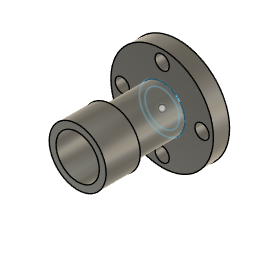
3D Plancha 1 (Autodesk Fusion 360 design; units mm, degrees)
Autodesk Fusion 360 part; units mm, degrees
sketch "Boceto1" plane through (0, 0, 0) normal (0, 1, 0) x (1, 0, 0)
  circle A0 centre (70, 0) radius 45
extrude "Extruir2" add sketch "Boceto1" along normal blind 14.2 makes body 1
sketch "Boceto2" plane through (0, 0, 0) normal (0, 1, 0) x (1, 0, 0)
  circle A0 centre (70, -35) radius 6.25
  circle A1 centre (35, 0) radius 6.25
  circle A2 centre (70, 35) radius 6.25
  circle A3 centre (105, 0) radius 6.25
extrude "Extruir3" cut sketch "Boceto2" along normal blind 15 bodies 1
sketch "Boceto3" plane through (0, 0, 0) normal (0, 1, 0) x (1, 0, 0)
  circle A0 centre (70, 0) radius 19
  circle A1 centre (70, 0) radius 24
  line L0 (70, -45) -> (70, -24)
  line L1 (70, -19) -> (70, 19)
  line L2 (70, 24) -> (70, 45)
  line L3 (25, 0) -> (46, 0)
  line L4 (51, 0) -> (89, 0)
  line L5 (94, 0) -> (115, 0)
  constraint horizontal L3
  constraint vertical L0
  constraint concentric A0 A1
  constraint coincident A1 L0.end
  constraint coincident A0 L1.start
  constraint collinear L0 L1
  constraint coincident A0.centre L0
  constraint coincident A0 L1.end
  constraint coincident A1 L2.start
  constraint collinear L1 L2
  constraint coincident A1 L3.end
  constraint coincident A0 L4.start
  constraint collinear L3 L4
  constraint coincident A0 L4.end
  constraint coincident A1 L5.start
  constraint collinear L4 L5
extrude "Extruir5" add sketch "Boceto3" against normal blind 44.2 bodies 1
sketch "Boceto7" plane through (0, 0, 0) normal (0, 1, 0) x (1, 0, 0)
  circle A0 centre (-25, 0) radius 25
  circle A1 centre (-25, 0) radius 19
  constraint concentric A0 A1
extrude "Extruir6" add sketch "Boceto7" against normal blind 30 separate body makes body 2
delete_face "SuprimirCaras2" 1 faces at (93.8807, -29.4667, 2.3896) on bodies 1
sketch "Boceto8" plane through (0, 0, 0) normal (0, 1, 0) x (1, 0, 0)
  circle A0 centre (70, 0) radius 15
  circle A1 centre (70, 0) radius 20
  constraint concentric A0 A1
extrude "Extruir7" add sketch "Boceto8" against normal blind 44.2 bodies 1
move_body "Alinear1" bodies 2 to x (1, 0, 0) y (0, 1, 0) z (0, 0, 1) at (95, -14.2, 0)
move_body "Desplazar1" bodies 2 to x (1, 0, 0) y (0, 1, 0) z (0, 0, 1) at (0, -30, 0)
combine "Combinar1" operation add target body 1 tool bodies 2
